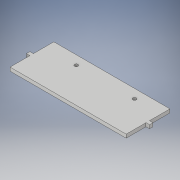
# Autodesk Inventor part: Lclamp2
Saved by Autodesk Inventor 2019 (Build 230136000, 136)
## iProperties
Created: 2020-02-26
Part Number: Lclamp2
Material: Generic
Document SubType Name: Modeling
Designer: Hp
Density: 1 g/cm^3
Appearance: Default
Author: Hp
Autodesk Inventor part; units mm, degrees
ref_plane "YZ Plane" through (0, 0, 0) normal (1, 0, 0) x (0, 1, 0)
ref_plane "XZ Plane" through (0, 0, 0) normal (0, 1, 0) x (-1, 0, 0)
ref_plane "XY Plane" through (0, 0, 0) normal (0, 0, 1) x (1, 0, 0)
sketch "Sketch1" plane through (0, 0, 0) normal (0, 1, 0) x (-1, 0, 0)
  line L0 (42.5071, 12.299) -> (-23.7769, 12.299)
  line L1 (-23.7769, 12.299) -> (-23.7769, -12.701)
  line L2 (-23.7769, -12.701) -> (42.5071, -12.701)
  line L3 (42.5071, -12.701) -> (42.5071, 12.299)
  line L4 (-23.7769, 0.9818) -> (-25.7769, 0.9818)
  line L5 (-25.7769, 0.9818) -> (-25.7769, -1.0182)
  line L6 (-25.7769, -1.0182) -> (-23.7769, -1.0182)
  line L7 (-23.7769, -1.0182) -> (-23.7769, 0.9818)
  line L8 (44.5071, -1.0182) -> (42.5071, -1.0182)
  line L9 (42.5071, -1.0182) -> (42.5071, 0.9818)
  line L10 (42.5071, 0.9818) -> (44.5071, 0.9818)
  line L11 (44.5071, 0.9818) -> (44.5071, -1.0182)
  point P0 (0, 0)
  dimension "d0" = 66.284
  dimension "d1" = 25
  dimension "d2" = 2
  dimension "d3" = 2
  dimension "d11" = 2
  dimension "d12" = 2
  constraints: 24 end point, 6 parallel, 3 horizontal, 3 perpendicular, 1 point on line
  measures "d0" distance of L2.end L1.end
  measures "d1" distance of L1.end L0.end
  measures "d2" distance of L6.end L5.end
  measures "d3" distance of L5.end L4.end
  measures "d11" distance of L9.end L10.end
  measures "d12" distance of L8.end L9.end
extrude "Extrusion1" add sketch "Sketch1" along normal blind 2
sketch "Sketch2" plane through (0, 2, 0) normal (0, 1, 0) x (1, 0, 0)
  circle A0 centre (8.7493, 7.4985) radius 1
  line L0 (8.7493, 7.4985) -> (-24.4607, 7.4985)
  circle A1 centre (-24.4607, 7.4985) radius 1
  point P0 (0, 0)
  dimension "d6" = 2
  dimension "d7" = 33.21
  dimension "d8" = 2
  constraints: 2 centre point, 2 end point, 1 coincident, 1 horizontal
  measures "d6" diameter of A0
  measures "d7" distance of L0.start L0.end
  measures "d8" diameter of A1
extrude "Extrusion2" cut sketch "Sketch2" against normal blind 2
body "Solid1"
